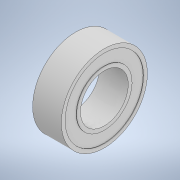
# Autodesk Inventor part: roller_5_9_3
Saved by Autodesk Inventor 2020 (Build 240168000, 168)
## iProperties
Created: 2024-02-24
Part Number: roller_5_9_3
Material: Типовые
Document SubType Name: Modeling
Designer: 4s
Density: 1 g/cm^3
Appearance: По умолчанию
Author: 4s
Autodesk Inventor part; units mm, degrees
ref_plane "YZ Plane" through (0, 0, 0) normal (1, 0, 0) x (0, 1, 0)
ref_plane "XZ Plane" through (0, 0, 0) normal (0, 1, 0) x (-1, 0, 0)
ref_plane "XY Plane" through (0, 0, 0) normal (0, 0, 1) x (1, 0, 0)
sketch "Эскиз1" plane through (0, 0, 0) normal (1, 0, 0) x (0, 1, 0)
  circle A0 centre (0, 0) radius 2.5
  circle A1 centre (0, 0) radius 4.5
  circle A2 centre (0, 0) radius 2.9
  circle A3 centre (0, 0) radius 4.1
  dimension "d0" = 5
  dimension "d1" = 9
  dimension "d2" = 0.4
  dimension "d3" = 0.4
  constraints: 4 centre point, 4 coincident
  measures "d0" diameter of A0
  measures "d1" diameter of A1
  measures "d2" radial gap between concentric circles of A1 A3
  measures "d3" radial gap between concentric circles of A2 A0
extrude "Выдавливание1" add sketch "Эскиз1" along normal mid plane 3
extrude "Выдавливание2" add sketch "Эскиз1" along normal mid plane 2.9 contours A3
